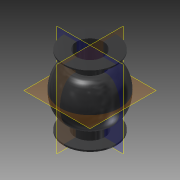
# Autodesk Inventor part: bump_black_small
Saved by Autodesk Inventor 2015 SP1 (Build 190203100, 203)
## iProperties
Created: 2015-07-16
Part Number: bump_black_small
Material: Rubber
Document SubType Name: Modeling
Designer: Alexandre Cherpillod
Density: 0.93 g/cm^3
Appearance: Rubber - Black - Version 1.1
Author: Alexandre Cherpillod
Autodesk Inventor part; units mm, degrees
sketch "Sketch5" plane through (0, 0, 0) normal (0, 1, 0) x (-1, 0, 0)
  line L0 (0, -8.4628) -> (0, 8.6242) projected
  ellipse E0 centre (2.8427, 0.0998) end of major axis (0.4846, 0.0998) minor radius 3.8913 (2.5, -3.7502) -> (2.5, 3.9498) ccw
  line L1 (2.5, -3.7502) -> (2.5, -5.7502)
  line L2 (2.5, -5.7502) -> (4.5, -5.7502)
  line L3 (2.5, 3.9498) -> (2.5, 5.9498)
  line L4 (2.5, 5.9498) -> (4.5, 5.9498)
  line L5 (4.5, 5.9498) -> (4.5, 6.1832)
  line L6 (4.5, 6.1832) -> (2.3, 6.1832)
  line L7 (2.3, 6.1832) -> (2.3, -6.0218)
  line L8 (2.3, -6.0218) -> (4.5, -6.0218)
  line L9 (4.5, -6.0218) -> (4.5, -5.7502)
  point P0 (0, 0)
  point P1 (5.2, -0.0087)
  dimension "d8" = 2
  dimension "d9" = 2
  dimension "d10" = 7.7
  dimension "d11" = 2.7
  dimension "d12" = 0.2
  dimension "d15" = 2.5
  constraints: 18 end point, 6 perpendicular, 3 vertical, 2 collinear, 1 point on line, 5 other
  measures "d8" distance of L1.start L1.end
  measures "d9" distance of L1.end L2.end
  measures "d10" distance of L3.start L1.start
  measures "d11" distance from line of L3 point (5.2, -0.009)
  measures "d12" distance between parallel lines of L7 L3
  measures "d15" distance between parallel lines of L0 L3
revolve "Revolution1" add sketch "Sketch5" angle 360 about axis through (0, 0, -10) along (0, 0, 1)
body "Solid1"
